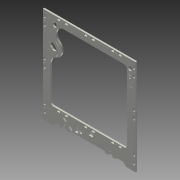
# Autodesk Inventor part: prawa_exp3
Saved by Autodesk Inventor 2013 (Build 170138000, 138)
## iProperties
Created: 2014-01-08
Part Number: prawa_exp3
Material: Generic
Document SubType Name: Modeling
Designer: dzban
Density: 1 g/cm^3
Author: dzban
Autodesk Inventor part; units mm, degrees
ref_plane "YZ Plane" through (0, 0, 0) normal (1, 0, 0) x (0, 1, 0)
ref_plane "XZ Plane" through (0, 0, 0) normal (0, 1, 0) x (-1, 0, 0)
ref_plane "XY Plane" through (0, 0, 0) normal (0, 0, 1) x (1, 0, 0)
sketch "Sketch1" plane through (0, 0, 0) normal (0, 1, 0) x (-1, 0, 0)
  arc A0 (5.6, 0.2) -> (5.6, 2.7) centre (5.6, 1.45) ccw
  line L0 (5.6, 0.2) -> (-0.4, 0.2)
  arc A1 (-0.4, 2.7) -> (-0.4, 0.2) centre (-0.4, 1.45) ccw
  line L1 (-0.4, 2.7) -> (5.6, 2.7)
  line L2 (-0.4, -6.8) -> (5.6, -6.8)
  arc A2 (5.6, -9.3) -> (5.6, -6.8) centre (5.6, -8.05) ccw
  line L3 (5.6, -9.3) -> (-0.4, -9.3)
  arc A3 (-0.4, -6.8) -> (-0.4, -9.3) centre (-0.4, -8.05) ccw
  line L4 (219.0652, -286.3311) -> (214.9513, -281.4284)
  line L5 (214.9513, -281.4284) -> (224.1439, -273.715)
  line L6 (224.1439, -273.715) -> (228.2577, -278.6176)
  line L7 (228.2577, -278.6176) -> (219.0652, -286.3311)
  line L8 (240.208, -268.5902) -> (236.0941, -263.6875)
  line L9 (236.0941, -263.6875) -> (245.2867, -255.974)
  line L10 (245.2867, -255.974) -> (249.4005, -260.8767)
  line L11 (249.4005, -260.8767) -> (240.208, -268.5902)
  line L12 (75.804, -281.7012) -> (75.804, -288.7012)
  line L13 (75.804, -288.7012) -> (81.904, -288.7012)
  line L14 (81.904, -288.7012) -> (82.204, -294.7012)
  line L15 (82.204, -294.7012) -> (94.004, -294.7012)
  line L16 (94.004, -294.7012) -> (94.304, -288.7012)
  line L17 (94.304, -288.7012) -> (176.8963, -288.7012)
  line L18 (176.8963, -288.7012) -> (177.1497, -288.7012)
  line L19 (177.1497, -288.7012) -> (178.1521, -288.7012)
  line L20 (178.1521, -288.7012) -> (224.304, -288.7012)
  line L21 (224.304, -288.7012) -> (224.604, -294.7012)
  line L22 (224.604, -294.7012) -> (236.404, -294.7012)
  line L23 (236.404, -294.7012) -> (236.704, -288.7012)
  line L24 (236.704, -288.7012) -> (242.804, -288.7012)
  line L25 (242.804, -288.7012) -> (242.804, -281.7012)
  line L26 (242.804, -281.7012) -> (241.554, -281.7012)
  line L27 (241.554, -281.7012) -> (241.554, -279.9012)
  line L28 (241.554, -279.9012) -> (242.804, -279.9012)
  line L29 (242.804, -279.9012) -> (242.804, -278.1012)
  line L30 (242.804, -278.1012) -> (245.804, -278.1012)
  line L31 (245.804, -278.1012) -> (245.804, -279.9012)
  line L32 (245.804, -279.9012) -> (247.054, -279.9012)
  line L33 (247.054, -279.9012) -> (247.054, -281.7012)
  line L34 (247.054, -281.7012) -> (245.804, -281.7012)
  line L35 (245.804, -281.7012) -> (245.804, -288.7012)
  line L36 (245.804, -288.7012) -> (251.904, -288.7012)
  line L37 (251.904, -288.7012) -> (252.204, -294.7012)
  line L38 (252.204, -294.7012) -> (264.004, -294.7012)
  line L39 (264.004, -294.7012) -> (264.304, -288.7012)
  line L40 (264.304, -288.7012) -> (273.4012, -288.7012)
  line L41 (273.4012, -288.7012) -> (284.7, -300)
  line L42 (284.7, -300) -> (324.7, -300)
  line L43 (324.7, -300) -> (324.7, 54.4)
  line L44 (324.7, 54.4) -> (-19.4, 54.4)
  line L45 (-19.4, 54.4) -> (-19.4, -300)
  line L46 (-19.4, -300) -> (15.6, -300)
  line L47 (15.6, -300) -> (26.8988, -288.7012)
  line L48 (26.8988, -288.7012) -> (54.304, -288.7012)
  line L49 (54.304, -288.7012) -> (54.604, -294.7012)
  line L50 (54.604, -294.7012) -> (66.404, -294.7012)
  line L51 (66.404, -294.7012) -> (66.704, -288.7012)
  line L52 (66.704, -288.7012) -> (72.804, -288.7012)
  line L53 (72.804, -288.7012) -> (72.804, -281.7012)
  line L54 (72.804, -281.7012) -> (71.554, -281.7012)
  line L55 (71.554, -281.7012) -> (71.554, -279.9012)
  line L56 (71.554, -279.9012) -> (72.804, -279.9012)
  line L57 (72.804, -279.9012) -> (72.804, -278.1012)
  line L58 (72.804, -278.1012) -> (75.804, -278.1012)
  line L59 (75.804, -278.1012) -> (75.804, -279.9012)
  line L60 (75.804, -279.9012) -> (77.054, -279.9012)
  line L61 (77.054, -279.9012) -> (77.054, -281.7012)
  line L62 (77.054, -281.7012) -> (75.804, -281.7012)
  line L63 (194.2359, -271.5554) -> (194.2359, -263.0554)
  line L64 (194.2359, -263.0554) -> (206.5359, -263.0554)
  line L65 (206.5359, -263.0554) -> (206.5359, -263.6804)
  arc A4 (159.35, -263.9049) -> (159.35, -256.0985) centre (146.85, -260.0017) ccw
  line L66 (206.5359, -271.4337) -> (206.5359, -282.3554)
  line L67 (206.5359, -282.3554) -> (194.2359, -282.3554)
  line L68 (194.2359, -282.3554) -> (194.2359, -274.3554)
  line L69 (194.2359, -274.3554) -> (191.5593, -274.3554)
  line L70 (191.5593, -274.3554) -> (191.5593, -271.5554)
  line L71 (191.5593, -271.5554) -> (194.2359, -271.5554)
  line L72 (-10, -0.4) -> (-16.4, -0.4)
  line L73 (-16.4, -0.4) -> (-16.4, 11.6)
  line L74 (-16.4, 11.6) -> (-10, 11.6)
  line L75 (-10, 11.6) -> (-10, -0.4)
  line L76 (-10, 27.2) -> (-16.4, 27.2)
  line L77 (-16.4, 27.2) -> (-16.4, 39.2)
  line L78 (-16.4, 39.2) -> (-10, 39.2)
  line L79 (-10, 39.2) -> (-10, 27.2)
  line L80 (-10, -135.4) -> (-16.4, -135.4)
  line L81 (-16.4, -135.4) -> (-16.4, -123.4)
  line L82 (-16.4, -123.4) -> (-10, -123.4)
  line L83 (-10, -123.4) -> (-10, -135.4)
  line L84 (-10, -107.8) -> (-16.4, -107.8)
  line L85 (-16.4, -107.8) -> (-16.4, -95.8)
  line L86 (-16.4, -95.8) -> (-10, -95.8)
  line L87 (-10, -95.8) -> (-10, -107.8)
  line L88 (-10, -279.8) -> (-16.4, -279.8)
  line L89 (-16.4, -279.8) -> (-16.4, -267.8)
  line L90 (-16.4, -267.8) -> (-10, -267.8)
  line L91 (-10, -267.8) -> (-10, -279.8)
  line L92 (-10, -252.2) -> (-16.4, -252.2)
  line L93 (-16.4, -252.2) -> (-16.4, -240.2)
  line L94 (-16.4, -240.2) -> (-10, -240.2)
  line L95 (-10, -240.2) -> (-10, -252.2)
  line L96 (315.3, -240.2) -> (321.7, -240.2)
  line L97 (321.7, -240.2) -> (321.7, -252.2)
  line L98 (321.7, -252.2) -> (315.3, -252.2)
  line L99 (315.3, -252.2) -> (315.3, -240.2)
  line L100 (315.3, -267.8) -> (321.7, -267.8)
  line L101 (321.7, -267.8) -> (321.7, -279.8)
  line L102 (321.7, -279.8) -> (315.3, -279.8)
  line L103 (315.3, -279.8) -> (315.3, -267.8)
  line L104 (315.3, -95.8) -> (321.7, -95.8)
  line L105 (321.7, -95.8) -> (321.7, -107.8)
  line L106 (321.7, -107.8) -> (315.3, -107.8)
  line L107 (315.3, -107.8) -> (315.3, -95.8)
  line L108 (315.3, -123.4) -> (321.7, -123.4)
  line L109 (321.7, -123.4) -> (321.7, -135.4)
  line L110 (321.7, -135.4) -> (315.3, -135.4)
  line L111 (315.3, -135.4) -> (315.3, -123.4)
  line L112 (315.3, 39.2) -> (321.7, 39.2)
  line L113 (321.7, 39.2) -> (321.7, 27.2)
  line L114 (321.7, 27.2) -> (315.3, 27.2)
  line L115 (315.3, 27.2) -> (315.3, 39.2)
  line L116 (315.3, 11.6) -> (321.7, 11.6)
  line L117 (321.7, 11.6) -> (321.7, -0.4)
  line L118 (321.7, -0.4) -> (315.3, -0.4)
  line L119 (315.3, -0.4) -> (315.3, 11.6)
  line L120 (232.85, -250) -> (232.85, -243.6)
  line L121 (232.85, -243.6) -> (244.85, -243.6)
  line L122 (244.85, -243.6) -> (244.85, -250)
  line L123 (244.85, -250) -> (232.85, -250)
  line L124 (260.45, -250) -> (260.45, -243.6)
  line L125 (260.45, -243.6) -> (272.45, -243.6)
  line L126 (272.45, -243.6) -> (272.45, -250)
  line L127 (272.45, -250) -> (260.45, -250)
  line L128 (132.85, -250) -> (132.85, -243.6)
  line L129 (132.85, -243.6) -> (144.85, -243.6)
  line L130 (144.85, -243.6) -> (144.85, -250)
  line L131 (144.85, -250) -> (132.85, -250)
  line L132 (160.45, -250) -> (160.45, -243.6)
  line L133 (160.45, -243.6) -> (172.45, -243.6)
  line L134 (172.45, -243.6) -> (172.45, -250)
  line L135 (172.45, -250) -> (160.45, -250)
  line L136 (32.85, -250) -> (32.85, -243.6)
  line L137 (32.85, -243.6) -> (44.85, -243.6)
  line L138 (44.85, -243.6) -> (44.85, -250)
  line L139 (44.85, -250) -> (32.85, -250)
  line L140 (60.45, -250) -> (60.45, -243.6)
  line L141 (60.45, -243.6) -> (72.45, -243.6)
  line L142 (72.45, -243.6) -> (72.45, -250)
  line L143 (72.45, -250) -> (60.45, -250)
  line L144 (232.85, 45) -> (232.85, 51.4)
  line L145 (232.85, 51.4) -> (244.85, 51.4)
  line L146 (244.85, 51.4) -> (244.85, 45)
  line L147 (244.85, 45) -> (232.85, 45)
  line L148 (260.45, 45) -> (260.45, 51.4)
  line L149 (260.45, 51.4) -> (272.45, 51.4)
  line L150 (272.45, 51.4) -> (272.45, 45)
  line L151 (272.45, 45) -> (260.45, 45)
  line L152 (132.85, 45) -> (132.85, 51.4)
  line L153 (132.85, 51.4) -> (144.85, 51.4)
  line L154 (144.85, 51.4) -> (144.85, 45)
  line L155 (144.85, 45) -> (132.85, 45)
  line L156 (160.45, 45) -> (160.45, 51.4)
  line L157 (160.45, 51.4) -> (172.45, 51.4)
  line L158 (172.45, 51.4) -> (172.45, 45)
  line L159 (172.45, 45) -> (160.45, 45)
  line L160 (32.85, 45) -> (32.85, 51.4)
  line L161 (32.85, 51.4) -> (44.85, 51.4)
  line L162 (44.85, 51.4) -> (44.85, 45)
  line L163 (44.85, 45) -> (32.85, 45)
  line L164 (60.45, 45) -> (60.45, 51.4)
  line L165 (60.45, 51.4) -> (72.45, 51.4)
  line L166 (72.45, 51.4) -> (72.45, 45)
  line L167 (72.45, 45) -> (60.45, 45)
  arc A5 (254.7, 16.4) -> (244.7, 26.4) centre (244.7, 16.4) ccw
  line L168 (254.7, 16.4) -> (254.7, -70.6)
  arc A6 (254.7, -70.6) -> (264.7, -80.6) centre (264.7, -70.6) ccw
  line L169 (264.7, -80.6) -> (286.7, -80.6)
  arc A7 (296.7, -90.6) -> (286.7, -80.6) centre (286.7, -90.6) ccw
  line L170 (296.7, -90.6) -> (296.7, -230.6)
  arc A8 (286.7, -240.6) -> (296.7, -230.6) centre (286.7, -230.6) ccw
  line L171 (286.7, -240.6) -> (22.6, -240.6)
  arc A9 (12.6, -230.6) -> (22.6, -240.6) centre (22.6, -230.6) ccw
  line L172 (12.6, -230.6) -> (12.6, 16.4)
  arc A10 (22.6, 26.4) -> (12.6, 16.4) centre (22.6, 16.4) ccw
  line L173 (22.6, 26.4) -> (244.7, 26.4)
  circle A11 centre (52.65, 48.2) radius 1.5
  circle A12 centre (152.65, 48.2) radius 1.5
  circle A13 centre (252.65, 48.2) radius 1.5
  circle A14 centre (52.65, -246.8) radius 1.5
  circle A15 centre (152.65, -246.8) radius 1.5
  circle A16 centre (252.65, -246.8) radius 1.5
  circle A17 centre (318.5, 19.4) radius 1.5
  circle A18 centre (318.5, -115.6) radius 1.5
  circle A19 centre (318.5, -260) radius 1.5
  circle A20 centre (-13.2, -260) radius 1.5
  circle A21 centre (-13.2, -115.6) radius 1.5
  circle A22 centre (-13.2, 19.4) radius 1.5
  circle A23 centre (185.1759, -272.7012) radius 6.25
  circle A24 centre (232.1759, -271.1526) radius 1.5
  circle A25 centre (2.3, 23.4) radius 8.05
  circle A26 centre (281.3, 12.4) radius 1.5
  circle A27 centre (2.3, 12.4) radius 1.5
  circle A28 centre (2.3, 34.4) radius 1.5
  circle A29 centre (281.3, 34.4) radius 1.5
  circle A30 centre (281.3, 23.4) radius 8.05
  circle A31 centre (1.6, -34.5124) radius 1.5
  circle A32 centre (-4.4, -34.5124) radius 1.5
  line L174 (206.5359, -271.4337) -> (206.5359, -263.6804)
  line L175 (140.85, -251.6228) -> (152.85, -251.6228)
  line L176 (154.85, -253.6228) -> (154.85, -265.6228)
  line L177 (152.85, -267.6228) -> (140.85, -267.6228)
  line L178 (138.85, -265.6228) -> (138.85, -253.6228)
  arc A33 (140.85, -251.6228) -> (138.85, -253.6228) centre (140.85, -253.6228) ccw
  arc A34 (154.85, -253.6228) -> (152.85, -251.6228) centre (152.85, -253.6228) ccw
  arc A35 (152.85, -267.6228) -> (154.85, -265.6228) centre (152.85, -265.6228) ccw
  arc A36 (138.85, -265.6228) -> (140.85, -267.6228) centre (140.85, -265.6228) ccw
  circle A37 centre (302.8, -64.1) radius 1.5
  point P0 (0, 0)
  point P1 (138.85, -251.6228)
  point P2 (154.85, -267.6228)
  point P3 (154.85, -251.6228)
  point P4 (138.85, -267.6228)
  dimension "d0" = 12
  dimension "d2" = 12
  dimension "d3" = 6.4
  dimension "d5" = 7.8
  dimension "d6" = 7.8
  dimension "d7" = 3.2
  dimension "d8" = 135
  dimension "d9" = 7.8
  dimension "d10" = 7.8
  dimension "d11" = 12
  dimension "d12" = 12
  dimension "d14" = 144.4
  dimension "d15" = 12
  dimension "d16" = 7.8
  dimension "d17" = 7.8
  dimension "d18" = 12
  dimension "d19" = 6.4
  dimension "d20" = 3.2
  dimension "d21" = 344.1
  dimension "d22" = 354.4
  dimension "d23" = 3
  dimension "d24" = 6.2
  dimension "d25" = 6.2
  dimension "d26" = 19.4
  dimension "d27" = 54.4
  dimension "d28" = 35
  dimension "d29" = 6.4
  dimension "d30" = 12
  dimension "d31" = 7.8
  dimension "d32" = 7.8
  dimension "d33" = 12
  dimension "d34" = 3.2
  dimension "d35" = 12
  dimension "d36" = 7.8
  dimension "d37" = 7.8
  dimension "d38" = 12
  dimension "d39" = 12
  dimension "d40" = 7.8
  dimension "d41" = 7.8
  dimension "d42" = 12
  dimension "d43" = 100
  dimension "d44" = 100
  dimension "d45" = 6.2
  dimension "d47" = 6.4
  dimension "d48" = 3.2
  dimension "d49" = 53.2
  dimension "d50" = 11
  dimension "d51" = 11
  dimension "d52" = 16.1
  dimension "d53" = 31
  dimension "d54" = 21.7
  dimension "d55" = 6
  dimension "d56" = 9.5
  dimension "d57" = 19
  dimension "d58" = 52.95
  dimension "d59" = 1.25
  dimension "d60" = 6
  dimension "d61" = 15
  dimension "d62" = 88.9125
  dimension "d63" = 43.4
  dimension "d74" = 11.2988
  dimension "d75" = 135
  dimension "d76" = 7
  dimension "d77" = 1.8
  constraints: 358 end point, 101 parallel, 90 collinear, 38 centre point, 30 point on circle, 26 tangent, 13 horizontal alignment, 13 vertical alignment, 12 equal radius, 8 point on line, 6 perpendicular, 2 horizontal
  measures "d0" distance between parallel lines of L74 L72
  measures "d2" distance between parallel lines of L78 L76
  measures "d3" distance between parallel lines of L77 L79
  measures "d5" distance from line of A22.centre L74
  measures "d6" distance from line of L76 A22.centre
  measures "d7" distance from line of L79 A22.centre
  measures "d8" distance of A22.centre A21.centre
  measures "d9" distance from line of L84 A21.centre
  measures "d10" distance from line of A21.centre L82
  measures "d11" distance between parallel lines of L82 L80
  measures "d12" distance between parallel lines of L86 L84
  measures "d14" distance of A20.centre A21.centre
  measures "d15" distance between parallel lines of L94 L92
  measures "d16" distance from line of L92 A20.centre
  measures "d17" distance from line of A20.centre L90
  measures "d18" distance between parallel lines of L90 L88
  measures "d19" distance between parallel lines of L113 L115
  measures "d20" distance from line of L113 A17.centre
  measures "d21" distance between parallel lines of L43 L45
  measures "d22" distance between parallel lines of L44 L46
  measures "d23" diameter of A22
  measures "d24" distance from line of L45 A22.centre
  measures "d25" distance from line of L43 A17.centre
  measures "d26" distance from line of L45 point (0, 0)
  measures "d27" distance from line of L44 point (0, 0)
  measures "d28" distance from line of L44 A22.centre
  measures "d29" distance between parallel lines of L161 L163
  measures "d30" distance between parallel lines of L162 L160
  measures "d31" distance from line of A11.centre L162
  measures "d32" distance from line of L164 A11.centre
  measures "d33" distance between parallel lines of L166 L164
  measures "d34" distance from line of L161 A11.centre
  measures "d35" distance between parallel lines of L154 L152
  measures "d36" distance from line of A12.centre L154
  measures "d37" distance from line of L156 A12.centre
  measures "d38" distance between parallel lines of L158 L156
  measures "d39" distance between parallel lines of L146 L144
  measures "d40" distance from line of A13.centre L146
  measures "d41" distance from line of L148 A13.centre
  measures "d42" distance between parallel lines of L150 L148
  measures "d43" distance of A12.centre A11.centre
  measures "d44" distance of A13.centre A12.centre
  measures "d45" distance from line of L44 A11.centre
  measures "d47" distance between parallel lines of L137 L139
  measures "d48" distance from line of A14.centre L139
  measures "d49" distance from line of L46 A14.centre
  measures "d50" distance of A28.centre A25.centre
  measures "d51" distance of A25.centre A27.centre
  measures "d52" diameter of A25
  measures "d53" distance from line of L44 A25.centre
  measures "d54" distance from line of L45 A25.centre
  measures "d55" distance of A0.centre A1.centre
  measures "d56" distance of A0.centre A2.centre
  measures "d57" distance from line of L45 A1.centre
  measures "d58" distance from line of L44 A1.centre
  measures "d59" radius of A0
  measures "d60" distance of A31.centre A32.centre
  measures "d61" distance from line of L45 A32.centre
  measures "d62" distance from line of L44 A32.centre
  measures "d63" distance from line of L43 A30.centre
  measures "d74" distance between parallel lines of L48 L46
  measures "d75" angle of L47 L46
  measures "d76" distance between parallel lines of L54 L52
  measures "d77" distance from line of L56 L54.end
extrude "Extrusion1" add sketch "Sketch1" along normal blind 6
sketch "Sketch2" plane through (0, 6, 0) normal (0, 1, 0) x (1, 0, 0)
  line L0 (-254.7, -16.4) -> (-254.7, 70.6) projected
  line L1 (-22.6, -26.4) -> (-244.7, -26.4) projected
  line L2 (-77.054, 281.7012) -> (-75.804, 281.7012) projected
  line L3 (-254.7, 21.6) -> (-266.7, 21.6)
  line L4 (-268.7, 19.6) -> (-268.7, 18.6)
  line L5 (-266.7, 16.6) -> (-254.7, 16.6)
  arc A0 (-266.7, 21.6) -> (-268.7, 19.6) centre (-266.7, 19.6) ccw
  arc A1 (-268.7, 18.6) -> (-266.7, 16.6) centre (-266.7, 18.6) ccw
  line L6 (-77.054, 279.9012) -> (-77.054, 281.7012) projected
  line L7 (-254.7, -9.9) -> (-260.7, -9.9)
  line L8 (-262.7, -11.9) -> (-262.7, -12.9)
  line L9 (-260.7, -14.9) -> (-254.7, -14.9)
  arc A2 (-260.7, -9.9) -> (-262.7, -11.9) centre (-260.7, -11.9) ccw
  arc A3 (-262.7, -12.9) -> (-260.7, -14.9) centre (-260.7, -12.9) ccw
  point P0 (0, 0)
  dimension "d145" = 5
  dimension "d147" = 43
  dimension "d148" = 14
  dimension "d149" = 2
  dimension "d196" = 5
  dimension "d197" = 31.5
  dimension "d198" = 8
  dimension "d199" = 2
  constraints: 12 end point, 8 point on circle, 8 tangent, 5 perpendicular, 4 centre point, 4 point on line, 2 equal radius, 1 parallel
  measures "d145" distance between parallel lines of L3 L5
  measures "d147" distance between parallel lines of L1 L5
  measures "d148" distance between parallel lines of L0 L4
  measures "d149" radius of A0
  measures "d196" distance between parallel lines of L7 L9
  measures "d197" distance between parallel lines of L3 L7
  measures "d198" distance between parallel lines of L0 L8
  measures "d199" radius of A2
extrude "Extrusion2" cut sketch "Sketch2" against normal blind 10
ref_plane "Work Plane1" through (-324.7, 0, 54.4) normal (-0.1736482, 0, 0.9848078) x (0, 1, 0)
sketch "Sketch6" plane through (0, 6, 0) normal (0, 1, 0) x (1, 0, 0)
  line L0 (-266.7, 21.6) -> (-254.7, 21.6) projected
  line L1 (-254.7, 21.6) -> (-254.7, 70.6) projected
  arc A0 (-254.7, 70.6) -> (-264.7, 80.6) centre (-264.7, 70.6) ccw projected
  line L2 (-264.7, 80.6) -> (-286.7, 80.6) projected
  arc A1 (-296.7, 90.6) -> (-286.7, 80.6) centre (-286.7, 90.6) ccw projected
  line L3 (-296.7, 90.6) -> (-296.7, 230.6) projected
  arc A2 (-286.7, 240.6) -> (-296.7, 230.6) centre (-286.7, 230.6) ccw projected
  line L4 (-286.7, 240.6) -> (-22.6, 240.6) projected
  arc A3 (-12.6, 230.6) -> (-22.6, 240.6) centre (-22.6, 230.6) ccw projected
  line L5 (-12.6, 230.6) -> (-12.6, -16.4) projected
  arc A4 (-22.6, -26.4) -> (-12.6, -16.4) centre (-22.6, -16.4) ccw projected
  line L6 (-22.6, -26.4) -> (-244.7, -26.4) projected
  arc A5 (-254.7, -16.4) -> (-244.7, -26.4) centre (-244.7, -16.4) ccw projected
  line L7 (-254.7, -16.4) -> (-254.7, 16.6) projected
  line L8 (-254.7, 16.6) -> (-266.7, 16.6) projected
  arc A6 (-268.7, 18.6) -> (-266.7, 16.6) centre (-266.7, 18.6) ccw projected
  line L9 (-268.7, 18.6) -> (-268.7, 19.6) projected
  arc A7 (-266.7, 21.6) -> (-268.7, 19.6) centre (-266.7, 19.6) ccw projected
  arc A8 (-154.85, 253.6228) -> (-152.85, 251.6228) centre (-152.85, 253.6228) ccw projected
  line L10 (-154.85, 253.6228) -> (-154.85, 265.6228) projected
  arc A9 (-152.85, 267.6228) -> (-154.85, 265.6228) centre (-152.85, 265.6228) ccw projected
  line L11 (-152.85, 267.6228) -> (-140.85, 267.6228) projected
  arc A10 (-138.85, 265.6228) -> (-140.85, 267.6228) centre (-140.85, 265.6228) ccw projected
  line L12 (-138.85, 265.6228) -> (-138.85, 253.6228) projected
  arc A11 (-140.85, 251.6228) -> (-138.85, 253.6228) centre (-140.85, 253.6228) ccw projected
  line L13 (-140.85, 251.6228) -> (-152.85, 251.6228) projected
  line L14 (-194.2359, 263.0554) -> (-206.5359, 263.0554) projected
  line L15 (-206.5359, 263.0554) -> (-206.5359, 282.3554) projected
  line L16 (-206.5359, 282.3554) -> (-194.2359, 282.3554) projected
  line L17 (-194.2359, 282.3554) -> (-194.2359, 274.3554) projected
  line L18 (-194.2359, 274.3554) -> (-191.5593, 274.3554) projected
  line L19 (-191.5593, 274.3554) -> (-191.5593, 271.5554) projected
  line L20 (-191.5593, 271.5554) -> (-194.2359, 271.5554) projected
  line L21 (-194.2359, 271.5554) -> (-194.2359, 263.0554) projected
  circle A12 centre (-281.3, -23.4) radius 8.05 projected
  circle A13 centre (-2.3, -23.4) radius 8.05 projected
  circle A14 centre (-185.1759, 272.7012) radius 6.25 projected
  line L22 (-60.45, -51.4) -> (-72.45, -51.4) projected
  line L23 (-72.45, -51.4) -> (-72.45, -45) projected
  line L24 (-72.45, -45) -> (-60.45, -45) projected
  line L25 (-60.45, -45) -> (-60.45, -51.4) projected
  line L26 (-32.85, -51.4) -> (-44.85, -51.4) projected
  line L27 (-44.85, -51.4) -> (-44.85, -45) projected
  line L28 (-44.85, -45) -> (-32.85, -45) projected
  line L29 (-32.85, -45) -> (-32.85, -51.4) projected
  line L30 (-160.45, -51.4) -> (-172.45, -51.4) projected
  line L31 (-172.45, -51.4) -> (-172.45, -45) projected
  line L32 (-172.45, -45) -> (-160.45, -45) projected
  line L33 (-160.45, -45) -> (-160.45, -51.4) projected
  line L34 (-132.85, -51.4) -> (-144.85, -51.4) projected
  line L35 (-144.85, -51.4) -> (-144.85, -45) projected
  line L36 (-144.85, -45) -> (-132.85, -45) projected
  line L37 (-132.85, -45) -> (-132.85, -51.4) projected
  line L38 (-260.45, -51.4) -> (-272.45, -51.4) projected
  line L39 (-272.45, -51.4) -> (-272.45, -45) projected
  line L40 (-272.45, -45) -> (-260.45, -45) projected
  line L41 (-260.45, -45) -> (-260.45, -51.4) projected
  line L42 (-232.85, -51.4) -> (-244.85, -51.4) projected
  line L43 (-244.85, -51.4) -> (-244.85, -45) projected
  line L44 (-244.85, -45) -> (-232.85, -45) projected
  line L45 (-232.85, -45) -> (-232.85, -51.4) projected
  line L46 (-60.45, 243.6) -> (-72.45, 243.6) projected
  line L47 (-72.45, 243.6) -> (-72.45, 250) projected
  line L48 (-72.45, 250) -> (-60.45, 250) projected
  line L49 (-60.45, 250) -> (-60.45, 243.6) projected
  line L50 (-32.85, 243.6) -> (-44.85, 243.6) projected
  line L51 (-44.85, 243.6) -> (-44.85, 250) projected
  line L52 (-44.85, 250) -> (-32.85, 250) projected
  line L53 (-32.85, 250) -> (-32.85, 243.6) projected
  line L54 (-160.45, 243.6) -> (-172.45, 243.6) projected
  line L55 (-172.45, 243.6) -> (-172.45, 250) projected
  line L56 (-172.45, 250) -> (-160.45, 250) projected
  line L57 (-160.45, 250) -> (-160.45, 243.6) projected
  line L58 (-132.85, 243.6) -> (-144.85, 243.6) projected
  line L59 (-144.85, 243.6) -> (-144.85, 250) projected
  line L60 (-144.85, 250) -> (-132.85, 250) projected
  line L61 (-132.85, 250) -> (-132.85, 243.6) projected
  line L62 (-260.45, 243.6) -> (-272.45, 243.6) projected
  line L63 (-272.45, 243.6) -> (-272.45, 250) projected
  line L64 (-272.45, 250) -> (-260.45, 250) projected
  line L65 (-260.45, 250) -> (-260.45, 243.6) projected
  line L66 (-232.85, 243.6) -> (-244.85, 243.6) projected
  line L67 (-244.85, 243.6) -> (-244.85, 250) projected
  line L68 (-244.85, 250) -> (-232.85, 250) projected
  line L69 (-232.85, 250) -> (-232.85, 243.6) projected
  line L70 (-321.7, -11.6) -> (-321.7, 0.4) projected
  line L71 (-321.7, 0.4) -> (-315.3, 0.4) projected
  line L72 (-315.3, 0.4) -> (-315.3, -11.6) projected
  line L73 (-315.3, -11.6) -> (-321.7, -11.6) projected
  line L74 (-321.7, -39.2) -> (-321.7, -27.2) projected
  line L75 (-321.7, -27.2) -> (-315.3, -27.2) projected
  line L76 (-315.3, -27.2) -> (-315.3, -39.2) projected
  line L77 (-315.3, -39.2) -> (-321.7, -39.2) projected
  line L78 (-321.7, 123.4) -> (-321.7, 135.4) projected
  line L79 (-321.7, 135.4) -> (-315.3, 135.4) projected
  line L80 (-315.3, 135.4) -> (-315.3, 123.4) projected
  line L81 (-315.3, 123.4) -> (-321.7, 123.4) projected
  line L82 (-321.7, 95.8) -> (-321.7, 107.8) projected
  line L83 (-321.7, 107.8) -> (-315.3, 107.8) projected
  line L84 (-315.3, 107.8) -> (-315.3, 95.8) projected
  line L85 (-315.3, 95.8) -> (-321.7, 95.8) projected
  line L86 (-321.7, 267.8) -> (-321.7, 279.8) projected
  line L87 (-321.7, 279.8) -> (-315.3, 279.8) projected
  line L88 (-315.3, 279.8) -> (-315.3, 267.8) projected
  line L89 (-315.3, 267.8) -> (-321.7, 267.8) projected
  line L90 (-321.7, 240.2) -> (-321.7, 252.2) projected
  line L91 (-321.7, 252.2) -> (-315.3, 252.2) projected
  line L92 (-315.3, 252.2) -> (-315.3, 240.2) projected
  line L93 (-315.3, 240.2) -> (-321.7, 240.2) projected
  line L94 (16.4, 252.2) -> (16.4, 240.2) projected
  line L95 (16.4, 240.2) -> (10, 240.2) projected
  line L96 (10, 240.2) -> (10, 252.2) projected
  line L97 (10, 252.2) -> (16.4, 252.2) projected
  line L98 (16.4, 279.8) -> (16.4, 267.8) projected
  line L99 (16.4, 267.8) -> (10, 267.8) projected
  line L100 (10, 267.8) -> (10, 279.8) projected
  line L101 (10, 279.8) -> (16.4, 279.8) projected
  line L102 (16.4, 107.8) -> (16.4, 95.8) projected
  line L103 (16.4, 95.8) -> (10, 95.8) projected
  line L104 (10, 95.8) -> (10, 107.8) projected
  line L105 (10, 107.8) -> (16.4, 107.8) projected
  line L106 (16.4, 135.4) -> (16.4, 123.4) projected
  line L107 (16.4, 123.4) -> (10, 123.4) projected
  line L108 (10, 123.4) -> (10, 135.4) projected
  line L109 (10, 135.4) -> (16.4, 135.4) projected
  line L110 (16.4, -27.2) -> (16.4, -39.2) projected
  line L111 (16.4, -39.2) -> (10, -39.2) projected
  line L112 (10, -39.2) -> (10, -27.2) projected
  line L113 (10, -27.2) -> (16.4, -27.2) projected
  line L114 (16.4, 0.4) -> (16.4, -11.6) projected
  line L115 (16.4, -11.6) -> (10, -11.6) projected
  line L116 (10, -11.6) -> (10, 0.4) projected
  line L117 (10, 0.4) -> (16.4, 0.4) projected
  line L118 (-236.0941, 263.6875) -> (-245.2867, 255.974) projected
  line L119 (-245.2867, 255.974) -> (-249.4005, 260.8767) projected
  line L120 (-249.4005, 260.8767) -> (-240.208, 268.5902) projected
  line L121 (-240.208, 268.5902) -> (-236.0941, 263.6875) projected
  line L122 (-214.9513, 281.4284) -> (-224.1439, 273.715) projected
  line L123 (-224.1439, 273.715) -> (-228.2577, 278.6176) projected
  line L124 (-228.2577, 278.6176) -> (-219.0652, 286.3311) projected
  line L125 (-219.0652, 286.3311) -> (-214.9513, 281.4284) projected
  arc A15 (-5.6, 9.3) -> (-5.6, 6.8) centre (-5.6, 8.05) ccw projected
  line L126 (-5.6, 9.3) -> (0.4, 9.3) projected
  arc A16 (0.4, 6.8) -> (0.4, 9.3) centre (0.4, 8.05) ccw projected
  line L127 (0.4, 6.8) -> (-5.6, 6.8) projected
  line L128 (-5.6, -0.2) -> (0.4, -0.2) projected
  arc A17 (0.4, -2.7) -> (0.4, -0.2) centre (0.4, -1.45) ccw projected
  line L129 (0.4, -2.7) -> (-5.6, -2.7) projected
  arc A18 (-5.6, -0.2) -> (-5.6, -2.7) centre (-5.6, -1.45) ccw projected
  circle A19 centre (-302.8, 64.1) radius 1.5 projected
  circle A20 centre (4.4, 34.5124) radius 1.5 projected
  circle A21 centre (-1.6, 34.5124) radius 1.5 projected
  circle A22 centre (-281.3, -34.4) radius 1.5 projected
  circle A23 centre (-2.3, -34.4) radius 1.5 projected
  circle A24 centre (-2.3, -12.4) radius 1.5 projected
  circle A25 centre (-281.3, -12.4) radius 1.5 projected
  circle A26 centre (-232.1759, 271.1526) radius 1.5 projected
  circle A27 centre (13.2, -19.4) radius 1.5 projected
  circle A28 centre (13.2, 115.6) radius 1.5 projected
  circle A29 centre (13.2, 260) radius 1.5 projected
  circle A30 centre (-318.5, 260) radius 1.5 projected
  circle A31 centre (-318.5, 115.6) radius 1.5 projected
  circle A32 centre (-318.5, -19.4) radius 1.5 projected
  circle A33 centre (-252.65, 246.8) radius 1.5 projected
  circle A34 centre (-152.65, 246.8) radius 1.5 projected
  circle A35 centre (-52.65, 246.8) radius 1.5 projected
  circle A36 centre (-252.65, -48.2) radius 1.5 projected
  circle A37 centre (-152.65, -48.2) radius 1.5 projected
  circle A38 centre (-52.65, -48.2) radius 1.5 projected
  line L130 (-75.804, 281.7012) -> (-75.804, 288.7012) projected
  line L131 (-75.804, 288.7012) -> (-81.904, 288.7012) projected
  line L132 (-81.904, 288.7012) -> (-82.204, 294.7012) projected
  line L133 (-82.204, 294.7012) -> (-94.004, 294.7012) projected
  line L134 (-94.004, 294.7012) -> (-94.304, 288.7012) projected
  line L135 (-94.304, 288.7012) -> (-176.8963, 288.7012) projected
  line L136 (-176.8963, 288.7012) -> (-177.1497, 288.7012) projected
  line L137 (-177.1497, 288.7012) -> (-178.1521, 288.7012) projected
  line L138 (-178.1521, 288.7012) -> (-224.304, 288.7012) projected
  line L139 (-224.304, 288.7012) -> (-224.604, 294.7012) projected
  line L140 (-224.604, 294.7012) -> (-236.404, 294.7012) projected
  line L141 (-236.404, 294.7012) -> (-236.704, 288.7012) projected
  line L142 (-236.704, 288.7012) -> (-242.804, 288.7012) projected
  line L143 (-242.804, 288.7012) -> (-242.804, 281.7012) projected
  line L144 (-242.804, 281.7012) -> (-241.554, 281.7012) projected
  line L145 (-241.554, 281.7012) -> (-241.554, 279.9012) projected
  line L146 (-241.554, 279.9012) -> (-242.804, 279.9012) projected
  line L147 (-242.804, 279.9012) -> (-242.804, 278.1012) projected
  line L148 (-242.804, 278.1012) -> (-245.804, 278.1012) projected
  line L149 (-245.804, 278.1012) -> (-245.804, 279.9012) projected
  line L150 (-245.804, 279.9012) -> (-247.054, 279.9012) projected
  line L151 (-247.054, 279.9012) -> (-247.054, 281.7012) projected
  line L152 (-247.054, 281.7012) -> (-245.804, 281.7012) projected
  line L153 (-245.804, 281.7012) -> (-245.804, 288.7012) projected
  line L154 (-245.804, 288.7012) -> (-251.904, 288.7012) projected
  line L155 (-251.904, 288.7012) -> (-252.204, 294.7012) projected
  line L156 (-252.204, 294.7012) -> (-264.004, 294.7012) projected
  line L157 (-264.004, 294.7012) -> (-264.304, 288.7012) projected
  line L158 (-264.304, 288.7012) -> (-273.4012, 288.7012) projected
  line L159 (-273.4012, 288.7012) -> (-284.7, 300) projected
  line L160 (-284.7, 300) -> (-324.7, 300) projected
  line L161 (-324.7, 300) -> (-324.7, -54.4) projected
  line L162 (-324.7, -54.4) -> (19.4, -54.4) projected
  line L163 (19.4, -54.4) -> (19.4, 300) projected
  line L164 (19.4, 300) -> (-15.6, 300) projected
  line L165 (-15.6, 300) -> (-26.8988, 288.7012) projected
  line L166 (-26.8988, 288.7012) -> (-54.304, 288.7012) projected
  line L167 (-54.304, 288.7012) -> (-54.604, 294.7012) projected
  line L168 (-54.604, 294.7012) -> (-66.404, 294.7012) projected
  line L169 (-66.404, 294.7012) -> (-66.704, 288.7012) projected
  line L170 (-66.704, 288.7012) -> (-72.804, 288.7012) projected
  line L171 (-72.804, 288.7012) -> (-72.804, 281.7012) projected
  line L172 (-72.804, 281.7012) -> (-71.554, 281.7012) projected
  line L173 (-71.554, 281.7012) -> (-71.554, 279.9012) projected
  line L174 (-71.554, 279.9012) -> (-72.804, 279.9012) projected
  line L175 (-72.804, 279.9012) -> (-72.804, 278.1012) projected
  line L176 (-72.804, 278.1012) -> (-75.804, 278.1012) projected
  line L177 (-75.804, 278.1012) -> (-75.804, 279.9012) projected
  line L178 (-75.804, 279.9012) -> (-77.054, 279.9012) projected
  line L179 (-77.054, 279.9012) -> (-77.054, 281.7012) projected
  line L180 (-77.054, 281.7012) -> (-75.804, 281.7012) projected
  point P0 (0, 0)
ref_plane "Work Plane2" through (-302.8, 6, -64.1) normal (-0.1736482, 0, 0.9848078) x (0, 1, 0)
sketch "Sketch7" plane through (-302.8, 6, -64.1) normal (-0.1736482, 0, 0.9848078) x (0, 1, 0)
  line L0 (0, 1.5) -> (0, -1.5) projected
  line L1 (-6, -1.5) -> (-6, 1.5) projected
  line L2 (-8.6152, -29.5) -> (4.0743, -29.5)
  line L3 (4.0743, -29.5) -> (4.0743, -32.5)
  line L4 (4.0743, -32.5) -> (-8.6152, -32.5)
  line L5 (-8.6152, -32.5) -> (-8.6152, -29.5)
  line L6 (-8.6152, 0) -> (5.1545, 0) construction
  point P0 (-6, -309.3306)
  dimension "d173" = 3
  dimension "d175" = 31
  dimension "d176" = 1.5
  constraints: 10 end point, 2 parallel, 2 perpendicular, 1 horizontal
  measures "d173" distance between parallel lines of L2 L4
  measures "d175" distance from line of L1.end L2
  measures "d176" distance from line of L1.end L6
revolve "Revolution1" cut sketch "Sketch7" angle 30 about axis through (-302.8, -2.6152, -64.1) along (0, 1, 0)
ref_plane "Work Plane4" through (-302.8, 6, -64.1) normal (-0.819152, 0, 0.5735764) x (0, 1, 0)
ref_plane "Work Plane3" through (-324.7, 0, 54.4) normal (-0.819152, 0, 0.5735764) x (0, 1, 0)
fillet "Fillet3" radius 1.4 4 edges at (-270.7937, 3, -58.4564) (-273.7482, 3, -58.9774) (-275.0791, 3, -74.1896) (-272.26, 3, -75.2157)
sketch "Sketch8" plane through (-302.8, 6, -64.1) normal (-0.819152, 0, 0.5735764) x (0, 1, 0)
  line L0 (-10.0833, -42.35) -> (9.5167, -42.35)
  line L1 (9.5167, -42.35) -> (9.5167, -45.35)
  line L2 (9.5167, -45.35) -> (-10.0833, -45.35)
  line L3 (-10.0833, -45.35) -> (-10.0833, -42.35)
  line L4 (0, 1.5) -> (0, -1.5) projected
  line L5 (-6, -1.5) -> (-6, 1.5) projected
  line L6 (-8.1968, 0) -> (5.0168, 0) construction
  point P0 (-6, -226.1866)
  dimension "d179" = 3
  dimension "d181" = 1.5
  dimension "d182" = 43.85
  constraints: 10 end point, 2 parallel, 2 perpendicular, 1 horizontal
  measures "d179" distance between parallel lines of L0 L2
  measures "d181" distance from line of L5.end L6
  measures "d182" distance from line of L0 L5.end
revolve "Revolution2" cut sketch "Sketch8" angle 30 about axis through (-302.8, -2.1968, -64.1) along (0, 1, 0)
ref_plane "Work Plane6" through (-302.8, 6, -64.1) normal (-0.9063078, 0, 0.4226183) x (0, 1, 0)
ref_plane "Work Plane5" through (-324.7, 0, 54.4) normal (-0.9063078, 0, 0.4226183) x (0, 1, 0)
sketch "Sketch9" plane through (-302.8, 6, -64.1) normal (-0.9063078, 0, 0.4226183) x (0, 1, 0)
  line L0 (0, 1.5) -> (0, -1.5) projected
  line L1 (-6, -1.5) -> (-6, 1.5) projected
  line L2 (-18.1343, -13) -> (19.853, -13)
  line L3 (19.853, -13) -> (19.853, -31)
  line L4 (19.853, -31) -> (-18.1343, -31)
  line L5 (-18.1343, -31) -> (-18.1343, -13)
  line L6 (-8.4875, 0) -> (15.1242, 0) construction
  point P0 (-6, -186.0631)
  dimension "d188" = 18
  dimension "d190" = 1.5
  dimension "d191" = 13
  constraints: 10 end point, 2 parallel, 2 perpendicular, 1 horizontal
  measures "d188" distance between parallel lines of L2 L4
  measures "d190" distance from line of L1.end L6
  measures "d191" distance between parallel lines of L6 L2
revolve "Revolution3" cut sketch "Sketch9" angle 55 about axis through (-302.8, -2.4875, -64.1) along (0, 1, 0) and the other way 15
fillet "Fillet4" radius 8 3 edges at (-289.9975, 3, -61.8426) (-300.5426, 3, -51.2975) (-297.4169, 3, -33.571)
fillet "Fillet5" radius 1.4 4 edges at (-261.6989, 3, -44.9343) (-264.4179, 3, -46.2021) (-276.7883, 3, -26.9515) (-278.509, 3, -29.4089)
sketch "Sketch11" plane through (0, 6, 0) normal (0, 1, 0) x (1, 0, 0)
  line L0 (-254.7, 21.6) -> (-254.7, 70.6) projected
  arc A0 (-296.7, 90.6) -> (-286.7, 80.6) centre (-286.7, 90.6) ccw projected
  line L1 (-22.6, -26.4) -> (-244.7, -26.4) projected
  line L2 (-324.7, 300) -> (-324.7, -54.4) projected
  line L3 (-324.7, -54.4) -> (19.4, -54.4) projected
  arc A1 (-265.449, 24.5896) -> (-289.2238, 80.9237) centre (-286.7, 48.8049) ccw
  arc A2 (-265.449, 24.5896) -> (-254.7, 30.5661) centre (-246.2479, 2.7101) ccw
  line L4 (-254.4822, 48.8049) -> (-227.3127, -19.4)
  line L5 (-254.4822, 48.8049) -> (-238.85, 79.4131)
  line L6 (-238.85, 79.4131) -> (-260.45, 96.4798)
  line L7 (-260.45, 96.4798) -> (-284.1762, 80.9237)
  point P0 (0, 0)
  dimension "d200" = 38
  dimension "d201" = 103.2049
  dimension "d202" = 64.4356
  dimension "d205" = 29.1101
  constraints: 8 end point, 8 point on circle, 2 centre point, 2 tangent, 1 point on line
  measures "d200" distance from line of A1.centre L2
  measures "d201" distance from line of A1.centre L3
  measures "d202" diameter of A1
  measures "d205" radius of A2
extrude "Extrusion5" cut sketch "Sketch11" against normal blind 10 contours A2 L4 A1 L0 | L0 A1 L4 A2 | A1 L7 L6 L5
sketch "Sketch12" plane through (0, 6, 0) normal (0, 1, 0) x (1, 0, 0)
  arc A0 (-254.7, 52.5448) -> (-281.498, 80.6) centre (-286.7, 48.8049) ccw projected
  line L0 (-281.498, 80.6) -> (-286.7, 80.6) projected
  arc A1 (-296.7, 90.6) -> (-286.7, 80.6) centre (-286.7, 90.6) ccw projected
  line L1 (-296.7, 90.6) -> (-296.7, 230.6) projected
  circle A2 centre (-266.7, 107.7206) radius 30
  line L2 (-296.7, 107.7206) -> (-304.7, 88.1102)
  line L3 (-304.7, 88.1102) -> (-288.4137, 74.6657)
  line L4 (-288.4137, 74.6657) -> (-276.3435, 79.3128)
  point P0 (0, 0)
  dimension "d206" = 60
  constraints: 6 end point, 3 point on circle, 2 tangent, 1 centre point, 1 point on line
  measures "d206" diameter of A2
extrude "Extrusion6" add sketch "Sketch12" against normal blind 6 contours A0 L0 A1 L1 A2
sketch "Sketch13" plane through (0, 6, 0) normal (0, 1, 0) x (1, 0, 0)
  arc A0 (-287.1342, 37.3496) -> (-272.271, 58.7169) centre (-302.8, 64.1) ccw projected
  line L0 (-299.0555, 42.8637) -> (-299.4284, 44.9785) projected
  line L1 (-283.6785, 60.7284) -> (-272.4007, 58.7398) projected
  line L2 (-272.2035, 58.705) -> (-272.271, 58.7169) projected
  circle A1 centre (-282.9529, 52.477) radius 8
  line L3 (-281.5637, 60.3555) -> (-278.0396, 61.3732)
  line L4 (-278.0396, 61.3732) -> (-273.7933, 59.1619)
  line L5 (-273.7933, 59.1619) -> (-273.2807, 58.895)
  line L6 (-273.2807, 58.895) -> (-272.2235, 58.7085)
  line L7 (-272.2235, 58.7085) -> (-271.1904, 52.8499)
  line L8 (-271.1904, 52.8499) -> (-276.0496, 48.4342)
  point P0 (0, 0)
  dimension "d210" = 16
  constraints: 12 end point, 3 point on circle, 3 point on line, 2 tangent, 1 centre point, 1 collinear, 1 parallel
  measures "d210" diameter of A1
extrude "Extrusion7" add sketch "Sketch13" against normal blind 6 contours A1 L1 L6 A0 | A0 L2 L7 L8 | L3 L4 L5 L1
sketch "Sketch15" plane through (0, 6, 0) normal (0, 1, 0) x (1, 0, 0)
  circle A0 centre (-281.3, -12.4) radius 1.5 projected
  circle A1 centre (-281.3, -34.4) radius 1.5 projected
  point P0 (0, 0)
extrude "Extrusion8" add sketch "Sketch15" against normal blind 6
sketch "Sketch16" plane through (0, 6, 0) normal (0, 1, 0) x (1, 0, 0)
  circle A0 centre (-281.3, -23.4) radius 8.05 projected
  circle A1 centre (-281.3, -35.4) radius 1.5
  circle A2 centre (-281.3, -11.4) radius 1.5
  point P0 (0, 0)
  dimension "d216" = 3
  dimension "d218" = 3
  dimension "d219" = 12
  dimension "d220" = 12
  constraints: 2 centre point, 2 vertical alignment
  measures "d216" diameter of A1
  measures "d218" diameter of A2
  measures "d219" distance of A0.centre A1.centre
  measures "d220" distance of A2.centre A0.centre
extrude "Extrusion9" cut sketch "Sketch16" against normal blind 6 contours A1 | A2
body "Solid1"
